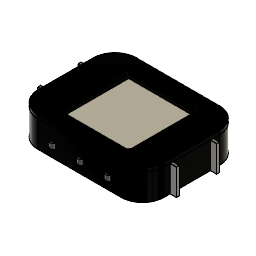
inktime_v6_cas (Autodesk Fusion 360 design; units mm, degrees)
part number: 2026-04-11-00-58-16-397
part number: 2026-04-11-00-58-25-501
part number: 2026-04-11-00-58-25-774
part number: 2026-04-11-00-58-25-861
part number: 2026-04-11-00-58-25-957
part number: 2026-04-11-00-58-26-614
part number: 2026-04-11-00-58-26-759
part number: 2026-04-11-00-58-26-889
part number: 2026-04-11-00-58-26-978
Autodesk Fusion 360 part; units mm, degrees
sketch "Sketch1" plane through (0, 0, 0) normal (0, 0, 1) x (1, 0, 0) in component "InkTime_Case"
  line L0 (-16.5, -19.5) -> (16.5, -19.5)
  line L1 (25, -11) -> (25, 11)
  line L2 (16.5, 19.5) -> (-16.5, 19.5)
  line L3 (-25, 11) -> (-25, -11)
  arc A0 (16.5, -19.5) -> (25, -11) centre (16.5, -11) ccw
  arc A1 (25, 11) -> (16.5, 19.5) centre (16.5, 11) ccw
  arc A2 (-16.5, 19.5) -> (-25, 11) centre (-16.5, 11) ccw
  arc A3 (-25, -11) -> (-16.5, -19.5) centre (-16.5, -11) ccw
  constraint tangent L0 A0
  constraint tangent L1 A0
  constraint tangent L1 A1
  constraint tangent L2 A1
  constraint tangent L2 A2
  constraint tangent L3 A2
  constraint tangent L3 A3
  constraint tangent L0 A3
extrude "Extrude1" add sketch "Sketch1" against normal blind 10.5 makes body 1 in component "InkTime_Case"
sketch "Sketch2" plane through (0, 0, 0) normal (0, 0, 1) x (1, 0, 0) in component "InkTime_Case"
  line L0 (-16.5, -18) -> (16.5, -18)
  line L1 (23.5, -11) -> (23.5, 11)
  line L2 (16.5, 18) -> (-16.5, 18)
  line L3 (-23.5, 11) -> (-23.5, -11)
  arc A0 (16.5, -18) -> (23.5, -11) centre (16.5, -11) ccw
  arc A1 (23.5, 11) -> (16.5, 18) centre (16.5, 11) ccw
  arc A2 (-16.5, 18) -> (-23.5, 11) centre (-16.5, 11) ccw
  arc A3 (-23.5, -11) -> (-16.5, -18) centre (-16.5, -11) ccw
  constraint tangent L0 A0
  constraint tangent L1 A0
  constraint tangent L1 A1
  constraint tangent L2 A1
  constraint tangent L2 A2
  constraint tangent L3 A2
  constraint tangent L3 A3
  constraint tangent L0 A3
extrude "Extrude2" cut sketch "Sketch2" against normal blind 9 bodies 1 in component "InkTime_Case"
sketch "Sketch3" plane through (0, 0, 0) normal (0, 0, 1) x (1, 0, 0) in component "InkTime_Case"
  line L0 (-16.5, -19.5) -> (16.5, -19.5)
  line L1 (25, -11) -> (25, 11)
  line L2 (16.5, 19.5) -> (-16.5, 19.5)
  line L3 (-25, 11) -> (-25, -11)
  arc A0 (16.5, -19.5) -> (25, -11) centre (16.5, -11) ccw
  arc A1 (25, 11) -> (16.5, 19.5) centre (16.5, 11) ccw
  arc A2 (-16.5, 19.5) -> (-25, 11) centre (-16.5, 11) ccw
  arc A3 (-25, -11) -> (-16.5, -19.5) centre (-16.5, -11) ccw
  constraint tangent L0 A0
  constraint tangent L1 A0
  constraint tangent L1 A1
  constraint tangent L2 A1
  constraint tangent L2 A2
  constraint tangent L3 A2
  constraint tangent L3 A3
  constraint tangent L0 A3
extrude "Extrude3" add sketch "Sketch3" along normal blind 1.5 separate body makes body 2 in component "InkTime_Case"
sketch "Sketch4" plane through (0, 0, 0) normal (0, 0, 1) x (1, 0, 0) in component "InkTime_Case"
  line L0 (-12.3, -13.8) -> (12.3, -13.8)
  line L1 (13.8, -12.3) -> (13.8, 12.3)
  line L2 (12.3, 13.8) -> (-12.3, 13.8)
  line L3 (-13.8, 12.3) -> (-13.8, -12.3)
  arc A0 (12.3, -13.8) -> (13.8, -12.3) centre (12.3, -12.3) ccw
  arc A1 (13.8, 12.3) -> (12.3, 13.8) centre (12.3, 12.3) ccw
  arc A2 (-12.3, 13.8) -> (-13.8, 12.3) centre (-12.3, 12.3) ccw
  arc A3 (-13.8, -12.3) -> (-12.3, -13.8) centre (-12.3, -12.3) ccw
  constraint tangent L0 A0
  constraint tangent L1 A0
  constraint tangent L1 A1
  constraint tangent L2 A1
  constraint tangent L2 A2
  constraint tangent L3 A2
  constraint tangent L3 A3
  constraint tangent L0 A3
extrude "Extrude4" cut sketch "Sketch4" along normal blind 2.5 bodies 2 in component "InkTime_Case"
ref_plane "WorkPlane1" through (0, 19.5, 0) normal (0, 1, 0) x (0, 0, 1) in component "InkTime_Case"
sketch "Sketch5" plane through (0, 19.5, 0) normal (0, 1, 0) x (1, 0, 0) in component "InkTime_Case"
ref_plane "WorkPlane2" through (0, -19.5, 0) normal (0, 1, 0) x (0, 0, 1) in component "InkTime_Case"
sketch "Sketch6" plane through (0, -19.5, 0) normal (0, 1, 0) x (1, 0, 0) in component "InkTime_Case"
sketch "Sketch1 (2)" plane through (0, 0, 0) normal (0, 0, 1) x (1, 0, 0) in component "Lug_Left"
  line L0 (-27.5, -8.6) -> (-25, -8.6)
  line L1 (-25, -8.6) -> (-25, -7.4)
  line L2 (-25, -7.4) -> (-27.5, -7.4)
  line L3 (-27.5, -7.4) -> (-27.5, -8.6)
extrude "Extrude1'" add sketch "Sketch1 (2)" against normal blind 10.5 separate body makes body 3 in component "Lug_Left"
sketch "Sketch2 (2)" plane through (0, 0, 0) normal (0, 0, 1) x (1, 0, 0) in component "Lug_Left"
  line L0 (-27.5, 7.4) -> (-25, 7.4)
  line L1 (-25, 7.4) -> (-25, 8.6)
  line L2 (-25, 8.6) -> (-27.5, 8.6)
  line L3 (-27.5, 8.6) -> (-27.5, 7.4)
extrude "Extrude2'" add sketch "Sketch2 (2)" against normal blind 10.5 separate body makes body 4 in component "Lug_Left"
sketch "Sketch1 (3)" plane through (0, 0, 0) normal (0, 0, 1) x (1, 0, 0) in component "Lug_Right"
  line L0 (25, -8.6) -> (27.5, -8.6)
  line L1 (27.5, -8.6) -> (27.5, -7.4)
  line L2 (27.5, -7.4) -> (25, -7.4)
  line L3 (25, -7.4) -> (25, -8.6)
extrude "Extrude1''" add sketch "Sketch1 (3)" against normal blind 10.5 separate body makes body 5 in component "Lug_Right"
sketch "Sketch2 (3)" plane through (0, 0, 0) normal (0, 0, 1) x (1, 0, 0) in component "Lug_Right"
  line L0 (25, 7.4) -> (27.5, 7.4)
  line L1 (27.5, 7.4) -> (27.5, 8.6)
  line L2 (27.5, 8.6) -> (25, 8.6)
  line L3 (25, 8.6) -> (25, 7.4)
extrude "Extrude2''" add sketch "Sketch2 (3)" against normal blind 10.5 separate body makes body 6 in component "Lug_Right"
sketch "Sketch1 (4)" plane through (0, 0, 0) normal (0, 0, 1) x (1, 0, 0) in component "InkTime_PCB"
  line L0 (-16, -17.5) -> (16, -17.5)
  line L1 (23, -10.5) -> (23, 10.5)
  line L2 (16, 17.5) -> (-16, 17.5)
  line L3 (-23, 10.5) -> (-23, -10.5)
  arc A0 (16, -17.5) -> (23, -10.5) centre (16, -10.5) ccw
  arc A1 (23, 10.5) -> (16, 17.5) centre (16, 10.5) ccw
  arc A2 (-16, 17.5) -> (-23, 10.5) centre (-16, 10.5) ccw
  arc A3 (-23, -10.5) -> (-16, -17.5) centre (-16, -10.5) ccw
  constraint tangent L0 A0
  constraint tangent L1 A0
  constraint tangent L1 A1
  constraint tangent L2 A1
  constraint tangent L2 A2
  constraint tangent L3 A2
  constraint tangent L3 A3
  constraint tangent L0 A3
extrude "Extrude1'''" add sketch "Sketch1 (4)" against normal blind 1.6 separate body makes body 7 in component "InkTime_PCB"
sketch "Sketch2 (4)" plane through (0, 0, 0) normal (0, 0, 1) x (1, 0, 0) in component "InkTime_PCB"
  line L0 (-24, -6.9) -> (-16, -6.9)
  line L1 (-16, -6.9) -> (-16, 6.9)
  line L2 (-16, 6.9) -> (-24, 6.9)
  line L3 (-24, 6.9) -> (-24, -6.9)
extrude "Extrude5" cut sketch "Sketch2 (4)" against normal blind 2.6 bodies 1 in component "InkTime_Case"
extrude "Extrude2'''" cut sketch "Sketch2 (4)" against normal blind 2.6 bodies 7 in component "InkTime_PCB"
sketch "Sketch3 (2)" plane through (0, 0, 0) normal (0, 0, 1) x (1, 0, 0) in component "InkTime_PCB"
  line L0 (-3.5, -5) -> (3.5, -5)
  line L1 (3.5, -5) -> (3.5, 2)
  line L2 (3.5, 2) -> (-3.5, 2)
  line L3 (-3.5, 2) -> (-3.5, -5)
extrude "Extrude3'" add sketch "Sketch3 (2)" along normal blind 0.8 separate body makes body 8 in component "InkTime_PCB"
sketch "Sketch4 (2)" plane through (0, 0, 0) normal (0, 0, 1) x (1, 0, 0) in component "InkTime_PCB"
  line L0 (-8, 2) -> (-6, 2)
  line L1 (-6, 2) -> (-6, 4)
  line L2 (-6, 4) -> (-8, 4)
  line L3 (-8, 4) -> (-8, 2)
extrude "Extrude4'" add sketch "Sketch4 (2)" along normal blind 0.5 separate body makes body 9 in component "InkTime_PCB"
sketch "Sketch5 (2)" plane through (0, 0, 0) normal (0, 0, 1) x (1, 0, 0) in component "InkTime_PCB"
  line L0 (-8, -6) -> (-6, -6)
  line L1 (-6, -6) -> (-6, -4)
  line L2 (-6, -4) -> (-8, -4)
  line L3 (-8, -4) -> (-8, -6)
extrude "Extrude5'" add sketch "Sketch5 (2)" along normal blind 0.5 separate body makes body 10 in component "InkTime_PCB"
sketch "Sketch6 (2)" plane through (0, 0, 0) normal (0, 0, 1) x (1, 0, 0) in component "InkTime_PCB"
  line L0 (14.4, 2.7) -> (17.6, 2.7)
  line L1 (17.6, 2.7) -> (17.6, 4.3)
  line L2 (17.6, 4.3) -> (14.4, 4.3)
  line L3 (14.4, 4.3) -> (14.4, 2.7)
extrude "Extrude6" add sketch "Sketch6 (2)" along normal blind 0.5 separate body makes body 11 in component "InkTime_PCB"
sketch "Sketch7" plane through (0, 0, 0) normal (0, 0, 1) x (1, 0, 0) in component "InkTime_PCB"
  line L0 (-10.5, 4.7) -> (-9.5, 4.7)
  line L1 (-9.5, 4.7) -> (-9.5, 5.3)
  line L2 (-9.5, 5.3) -> (-10.5, 5.3)
  line L3 (-10.5, 5.3) -> (-10.5, 4.7)
extrude "Extrude7" add sketch "Sketch7" along normal blind 0.3 separate body makes body 12 in component "InkTime_PCB"
sketch "Sketch8" plane through (0, 0, 0) normal (0, 0, 1) x (1, 0, 0) in component "InkTime_PCB"
  line L0 (9.5, 7.7) -> (10.5, 7.7)
  line L1 (10.5, 7.7) -> (10.5, 8.3)
  line L2 (10.5, 8.3) -> (9.5, 8.3)
  line L3 (9.5, 8.3) -> (9.5, 7.7)
extrude "Extrude8" add sketch "Sketch8" along normal blind 0.3 separate body makes body 13 in component "InkTime_PCB"
sketch "Sketch9" plane through (0, 0, 0) normal (0, 0, 1) x (1, 0, 0) in component "InkTime_PCB"
  line L0 (-8.5, -8.3) -> (-7.5, -8.3)
  line L1 (-7.5, -8.3) -> (-7.5, -7.7)
  line L2 (-7.5, -7.7) -> (-8.5, -7.7)
  line L3 (-8.5, -7.7) -> (-8.5, -8.3)
extrude "Extrude9" add sketch "Sketch9" along normal blind 0.3 separate body makes body 14 in component "InkTime_PCB"
sketch "Sketch10" plane through (0, 0, 0) normal (0, 0, 1) x (1, 0, 0) in component "InkTime_PCB"
  line L0 (11.5, -3.3) -> (12.5, -3.3)
  line L1 (12.5, -3.3) -> (12.5, -2.7)
  line L2 (12.5, -2.7) -> (11.5, -2.7)
  line L3 (11.5, -2.7) -> (11.5, -3.3)
extrude "Extrude10" add sketch "Sketch10" along normal blind 0.3 separate body makes body 15 in component "InkTime_PCB"
sketch "Sketch11" plane through (0, 0, 0) normal (0, 0, 1) x (1, 0, 0) in component "InkTime_PCB"
  line L0 (-5.5, 9.7) -> (-4.5, 9.7)
  line L1 (-4.5, 9.7) -> (-4.5, 10.3)
  line L2 (-4.5, 10.3) -> (-5.5, 10.3)
  line L3 (-5.5, 10.3) -> (-5.5, 9.7)
extrude "Extrude11" add sketch "Sketch11" along normal blind 0.3 separate body makes body 16 in component "InkTime_PCB"
sketch "Sketch12" plane through (0, 0, 0) normal (0, 0, 1) x (1, 0, 0) in component "InkTime_PCB"
  line L0 (7.5, -10.3) -> (8.5, -10.3)
  line L1 (8.5, -10.3) -> (8.5, -9.7)
  line L2 (8.5, -9.7) -> (7.5, -9.7)
  line L3 (7.5, -9.7) -> (7.5, -10.3)
extrude "Extrude12" add sketch "Sketch12" along normal blind 0.3 separate body makes body 17 in component "InkTime_PCB"
move_body "Move1" bodies 7 8 9 10 11 12 13 14 15 16 17 to x (1, 0, 0) y (0, 1, 0) z (0, 0, 1) at (0, 0, -5) in component "InkTime_PCB"
sketch "Sketch1 (5)" plane through (0, 0, 0) normal (0, 0, 1) x (1, 0, 0) in component "InkTime_EPaper"
  line L0 (-15.5, -18.5) -> (15.5, -18.5)
  line L1 (15.5, -18.5) -> (15.5, 18.5)
  line L2 (15.5, 18.5) -> (-15.5, 18.5)
  line L3 (-15.5, 18.5) -> (-15.5, -18.5)
extrude "Extrude1''''" add sketch "Sketch1 (5)" against normal blind 1.2 separate body makes body 18 in component "InkTime_EPaper"
sketch "Sketch2 (5)" plane through (0, 0, 0) normal (0, 0, 1) x (1, 0, 0) in component "InkTime_EPaper"
  line L0 (-13.8, -13.8) -> (13.8, -13.8)
  line L1 (13.8, -13.8) -> (13.8, 13.8)
  line L2 (13.8, 13.8) -> (-13.8, 13.8)
  line L3 (-13.8, 13.8) -> (-13.8, -13.8)
extrude "Extrude2''''" add sketch "Sketch2 (5)" along normal blind 0.15 separate body makes body 19 in component "InkTime_EPaper"
move_body "Move1'" bodies 18 19 to x (1, 0, 0) y (0, 1, 0) z (0, 0, 1) at (0, 0, -1.5) in component "InkTime_EPaper"
sketch "Sketch1 (6)" plane through (0, 0, 0) normal (0, 0, 1) x (1, 0, 0) in component "InkTime_Battery"
  line L0 (-11, -10) -> (11, -10)
  line L1 (15, -6) -> (15, 6)
  line L2 (11, 10) -> (-11, 10)
  line L3 (-15, 6) -> (-15, -6)
  arc A0 (11, -10) -> (15, -6) centre (11, -6) ccw
  arc A1 (15, 6) -> (11, 10) centre (11, 6) ccw
  arc A2 (-11, 10) -> (-15, 6) centre (-11, 6) ccw
  arc A3 (-15, -6) -> (-11, -10) centre (-11, -6) ccw
  constraint tangent L0 A0
  constraint tangent L1 A0
  constraint tangent L1 A1
  constraint tangent L2 A1
  constraint tangent L2 A2
  constraint tangent L3 A2
  constraint tangent L3 A3
  constraint tangent L0 A3
extrude "Extrude1'''''" add sketch "Sketch1 (6)" against normal blind 3.5 separate body makes body 20 in component "InkTime_Battery"
move_body "Move1''" bodies 20 to x (1, 0, 0) y (0, 1, 0) z (0, 0, 1) at (0, 0, -5.2) in component "InkTime_Battery"
sketch "Sketch1 (7)" plane through (0, 0, 0) normal (0, 0, 1) x (1, 0, 0) in component "InkTime_Motor"
  circle A0 centre (-6, -2) radius 5
extrude "Extrude1''''''" add sketch "Sketch1 (7)" against normal blind 2.7 separate body makes body 21 in component "InkTime_Motor"
move_body "Move1'''" bodies 21 to x (1, 0, 0) y (0, 1, 0) z (0, 0, 1) at (0, 0, -3.1) in component "InkTime_Motor"
sketch "Sketch1 (8)" plane through (0, 0, 0) normal (0, 0, 1) x (1, 0, 0) in component "InkTime_Buttons"
  circle A0 centre (-11, -18.75) radius 1.3
extrude "Extrude1'''''''" add sketch "Sketch1 (8)" against normal blind 2 separate body makes body 22 in component "InkTime_Buttons"
sketch "Sketch2 (6)" plane through (0, 0, 0) normal (0, 0, 1) x (1, 0, 0) in component "InkTime_Buttons"
  circle A0 centre (0, -18.75) radius 1.3
extrude "Extrude2'''''" add sketch "Sketch2 (6)" against normal blind 2 separate body makes body 23 in component "InkTime_Buttons"
sketch "Sketch3 (3)" plane through (0, 0, 0) normal (0, 0, 1) x (1, 0, 0) in component "InkTime_Buttons"
  circle A0 centre (11, -18.75) radius 1.3
extrude "Extrude3''" add sketch "Sketch3 (3)" against normal blind 2 separate body makes body 24 in component "InkTime_Buttons"
move_body "Move1''''" bodies 22 23 24 to x (1, 0, 0) y (0, 1, 0) z (0, 0, 1) at (0, 0, -5.25) in component "InkTime_Buttons"
sketch "Sketch1 (9)" plane through (0, 19.5, 0) normal (0, 1, 0) x (-1, 0, 0)
  line L0 (16.5, 0) -> (-16.5, 0)
  line L1 (-16.5, 0) -> (-16.5, -10.5)
  line L2 (-16.5, -10.5) -> (16.5, -10.5)
  line L3 (16.5, -10.5) -> (16.5, 0)
  line L4 (-6, -2.8279) -> (6.058, -2.8279)
  line L5 (6.058, -2.8279) -> (6.058, -6.079)
  line L6 (6.058, -6.079) -> (-6, -6.079)
  line L7 (-6, -6.079) -> (-6, -2.8279)
  constraint horizontal L4
  constraint vertical L5
  constraint horizontal L6
  constraint vertical L7
extrude "Extrude6'" add sketch "Sketch1 (9)" along normal blind 1.5 contours L4 L5 L6 L7 bodies 1 in component "InkTime_Case"
extrude "Extrude7'" cut 1 faces at (1.9807, 21, -3.9116) along direction (0, -1, 0) blind 0.5 on bodies 1 bodies 1 in component "InkTime_Case"
extrude "Extrude8'" cut 1 faces at (1.9807, 20.5, -3.9116) along direction (0, -1, 0) blind 0.2 on bodies 1 bodies 1 in component "InkTime_Case"
extrude "Extrude9'" cut 1 faces at (1.9807, 20.3, -3.9116) along direction (0, -1, 0) blind 2.5 on bodies 1 bodies 1 in component "InkTime_Case"
fillet "Fillet1" radius 1 1 edges at (-6.058, 18.75, -6.079) on bodies 1 in component "InkTime_Case"
fillet "Fillet2" radius 1 1 edges at (6, 18.75, -6.079) on bodies 1 in component "InkTime_Case"
fillet "Fillet3" radius 1 1 edges at (6, 18.75, -2.8279) on bodies 1 in component "InkTime_Case"
fillet "Fillet4" radius 1 1 edges at (-6.058, 18.75, -2.8279) on bodies 1 in component "InkTime_Case"
component "InkTime_Case" placed x (1, 0, 0) y (0, 1, 0) z (0, 0, 1) at (0, 0, 0)
component "Lug_Left" placed x (1, 0, 0) y (0, 1, 0) z (0, 0, 1) at (0, 0, 0)
component "Lug_Right" placed x (1, 0, 0) y (0, 1, 0) z (0, 0, 1) at (0, 0, 0)
component "InkTime_PCB" placed x (1, 0, 0) y (0, 1, 0) z (0, 0, 1) at (0, 0, 0)
component "InkTime_EPaper" placed x (1, 0, 0) y (0, 1, 0) z (0, 0, 1) at (0, 0, 0)
component "InkTime_Battery" placed x (1, 0, 0) y (0, 1, 0) z (0, 0, 1) at (0, 0, 0)
component "InkTime_Motor" placed x (1, 0, 0) y (0, 1, 0) z (0, 0, 1) at (0, 0, 0)
component "InkTime_Buttons" placed x (1, 0, 0) y (0, 1, 0) z (0, 0, 1) at (0, 0, 0)
equation "d1 = -( 10.50 mm )"
equation "d3 = -( 9.00 mm )"
equation "d11 = -( 10.50 mm )"
equation "d13 = -( 10.50 mm )"
equation "d15 = -( 10.50 mm )"
equation "d17 = -( 10.50 mm )"
equation "d19 = -( 1.60 mm )"
equation "d21 = -( 2.60 mm )"
equation "d23 = -( 2.60 mm )"
equation "d45 = -( 1.20 mm )"
equation "d49 = -( 3.50 mm )"
equation "d51 = -( 2.70 mm )"
equation "d53 = -( 2.00 mm )"
equation "d55 = -( 2.00 mm )"
equation "d57 = -( 2.00 mm )"
named bodies: "Case", "Bezel", "PCB_FR4", "nRF52840", "BQ25180", "RT6160", "ANT1", "SMD_C1", "SMD_C2", "SMD_R1", "SMD_L3", "SMD_IC3", "SMD_C3", "EPaper_PCB", "EPaper_Screen", "LiPo_Pouch", "Motor", "SW_ENT", "SW_DN", "SW_UP"
